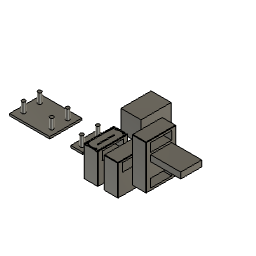
Scintillator Fittings (Autodesk Fusion 360 design; units mm, degrees)
Autodesk Fusion 360 part; units mm, degrees
note: some values were not read from the file. Set by a fixed rule: which sketch regions a step uses.
sketch "Sketch1" plane through (0, 0, 0) normal (0, 0, 1) x (1, 0, 0)
  line L0 (17.5, 37.5) -> (-17.5, 37.5)
  line L1 (-17.5, 37.5) -> (-17.5, -37.5)
  line L2 (-17.5, -37.5) -> (17.5, -37.5)
  line L3 (17.5, -37.5) -> (17.5, 37.5)
  line L4 (17.5, 37.5) -> (-17.5, -37.5) construction
  line L5 (-17.5, 37.5) -> (17.5, -37.5) construction
  dimension "d1" = 35
  dimension "d2" = 75
  constraint horizontal L0
  constraint perpendicular L0 L1
  constraint parallel L0 L2
  constraint parallel L1 L3
  constraint coincident L4 origin
  constraint coincident L5 origin
  measures "d1" distance of L1.end L2.end
  measures "d2" distance of L0.end L1.end
extrude "Extrude1" add sketch "Sketch1" along normal blind 5 makes body 1
sketch "Sketch2" plane through (0, 0, 5) normal (0, 0, 1) x (-1, 0, 0)
  line L0 (-17.5, 37.5) -> (-17.5, -37.5)
  line L1 (-17.5, -37.5) -> (17.5, -37.5)
  line L2 (17.5, -37.5) -> (17.5, 37.5)
  line L3 (17.5, 37.5) -> (-17.5, 37.5)
  line L4 (-17.5, -26.25) -> (17.5, -26.25)
  line L5 (17.5, -26.25) -> (17.5, 26.25)
  line L6 (17.5, 26.25) -> (-17.5, 26.25)
  line L7 (-17.5, 26.25) -> (-17.5, -26.25)
  line L8 (-17.5, -26.25) -> (17.5, 26.25) construction
  line L9 (17.5, -26.25) -> (-17.5, 26.25) construction
  dimension "d5" = 52.5
  constraint horizontal L4
  constraint perpendicular L4 L5
  constraint parallel L4 L6
  constraint parallel L5 L7
  constraint coincident L8 origin
  constraint coincident L9 origin
  measures "d5" distance of L4.end L5.end
extrude "Extrude2" add sketch "Sketch2" along normal blind 26 contours L0 L2 L3 L6 | L0 L1 L2 L4 bodies 1
sketch "Sketch3" plane through (0, -26.25, 0) normal (0, 1, 0) x (-1, 0, 0)
  line L0 (-17.5, 5) -> (17.5, 5)
  line L1 (17.5, 5) -> (17.5, 31)
  line L2 (17.5, 31) -> (-17.5, 31)
  line L3 (-17.5, 31) -> (-17.5, 5)
  line L4 (-17.5, 31) -> (17.5, 31)
  line L5 (17.5, 31) -> (17.5, 26)
  line L6 (17.5, 26) -> (-17.5, 26)
  line L7 (-17.5, 26) -> (-17.5, 31)
  dimension "d8" = 35
  dimension "d9" = 5
  constraint horizontal L4
  constraint vertical L5
  constraint horizontal L6
  constraint vertical L7
  constraint coincident L2.end L3.start
  measures "d8" distance of L2.end L1.end
  measures "d9" distance of L2.end L6.end
extrude "Extrude3" add sketch "Sketch3" along normal blind 52.5 contours L1 L2 L3 L4 L5 L6 L7 bodies 1
chamfer "Chamfer1" distance 1 angle 45 8 edges at (0, -37.5, 31) (17.5, 0, 31) (-17.5, 0, 31) (0, 37.5, 31) (17.5, 37.5, 15.5) (-17.5, 37.5, 15.5) (-17.5, -37.5, 15.5) (17.5, -37.5, 15.5) on bodies 1
sketch "Sketch4" plane through (0, 0, 31) normal (0, 0, 1) x (-1, 0, 0)
  line L0 (-16.5, 36.5) -> (-16.5, -36.5)
  line L1 (-16.5, -36.5) -> (16.5, -36.5)
  line L2 (16.5, -36.5) -> (16.5, 36.5)
  line L3 (16.5, 36.5) -> (-16.5, 36.5)
  line L4 (-16, 20) -> (-16, -20)
  line L5 (16, -20) -> (16, 20)
  line L6 (16, 20) -> (-16, -20) construction
  line L7 (-16, 20) -> (16, -20) construction
  circle A0 centre (0, -20) radius 16
  circle A1 centre (0, 20) radius 16
  dimension "d13" = 32
  dimension "d14" = 40
  dimension "d15" = 32
  dimension "d16" = 32
  constraint parallel L4 L5
  constraint coincident L6 origin
  constraint coincident L7 origin
  measures "d13" distance of L4.end L5.start
  measures "d14" distance of L4.start L4.end
  measures "d15" diameter of A0
  measures "d16" diameter of A1
extrude "Extrude4" cut sketch "Sketch4" against normal blind 2.5 contours L4 L5 A0 A1 | A1 | A0 bodies 1
sketch "Sketch5" plane through (0, 0, 28.5) normal (0, 0, 1) x (-1, 0, 0)
  arc A0 (16, 20) -> (-16, 20) centre (0, 20) ccw
  line L0 (-16, 20) -> (-16, -20)
  arc A1 (-16, -20) -> (16, -20) centre (0, -20) ccw
  line L1 (16, -20) -> (16, 20)
  circle A2 centre (0, -20) radius 1.25
  circle A3 centre (0, 20) radius 1.25
  line L2 (-1.25, -20) -> (-1.25, 20)
  line L3 (1.25, 20) -> (1.25, -20)
  line L4 (1.25, -20) -> (-1.25, 20) construction
  line L5 (-1.25, -20) -> (1.25, 20) construction
  dimension "d19" = 2.5
  dimension "d20" = 2.5
  dimension "d21" = 2.5
  dimension "d22" = 40
  constraint concentric A1 A2
  constraint concentric A0 A3
  constraint parallel L2 L3
  constraint coincident L4 origin
  constraint coincident L5 origin
  measures "d19" diameter of A2
  measures "d20" diameter of A3
  measures "d21" distance of L2.end L3.start
  measures "d22" distance of L2.start L2.end
extrude "Extrude5" cut sketch "Sketch5" against normal blind 2.5 contours A2 | A2 A3 L2 L3 | A3 bodies 1
sketch "Sketch6" plane through (0, 0, 31) normal (0, 0, 1) x (-1, 0, 0)
  line L0 (-16, -20) -> (-16, 20)
  arc A0 (16, 20) -> (-16, 20) centre (0, 20) ccw
  line L1 (16, 20) -> (16, -20)
  arc A1 (-16, -20) -> (16, -20) centre (0, -20) ccw
  line L2 (-16.5, 36.5) -> (-16.5, -36.5)
  line L3 (-16.5, -36.5) -> (16.5, -36.5)
  line L4 (16.5, -36.5) -> (16.5, 36.5)
  line L5 (16.5, 36.5) -> (-16.5, 36.5)
  line L6 (-15, -37.5) -> (15, -37.5)
  line L7 (15, -37.5) -> (15, 37.5)
  line L8 (15, 37.5) -> (-15, 37.5)
  line L9 (-15, 37.5) -> (-15, -37.5)
  line L10 (-15, -37.5) -> (15, 37.5) construction
  line L11 (15, -37.5) -> (-15, 37.5) construction
  line L12 (-10, 37.5) -> (10, 37.5)
  line L13 (10, 37.5) -> (10, -37.5)
  line L14 (10, -37.5) -> (-10, -37.5)
  line L15 (-10, -37.5) -> (-10, 37.5)
  line L16 (-10, 37.5) -> (10, -37.5) construction
  line L17 (10, 37.5) -> (-10, -37.5) construction
  dimension "d25" = 30
  dimension "d26" = 75
  dimension "d27" = 20
  dimension "d28" = 75
  constraint horizontal L6
  constraint perpendicular L6 L7
  constraint parallel L6 L8
  constraint parallel L7 L9
  constraint coincident L10 origin
  constraint coincident L11 origin
  constraint horizontal L12
  constraint perpendicular L12 L13
  constraint parallel L12 L14
  constraint parallel L13 L15
  constraint coincident L16 origin
  constraint coincident L17 origin
  measures "d25" distance of L7.end L8.end
  measures "d26" distance of L6.end L7.end
  measures "d27" distance of L13.end L14.end
  measures "d28" distance of L12.end L13.end
extrude "Extrude6" cut sketch "Sketch6" against normal blind 2.5 contours A1 L3 L9 L15 | A0 L5 L9 L15 | L3 L6 L9 L15 | L5 L8 L9 L15 | A1 L3 L7 L13 | A0 L5 L7 L13 | L3 L6 L7 L13 | L5 L7 L8 L13 bodies 1
chamfer "Chamfer2" distance 0.5 angle 45 8 edges at (-10, -34.495, 31) (10, -34.495, 31) (15, -31.0339, 31) (-15, -31.0339, 31) (-10, 34.495, 31) (-15, 31.0339, 31) (10, 34.495, 31) (15, 31.0339, 31) on bodies 1
sketch "Sketch7" plane through (0, 0, 0) normal (0, 0, 1) x (1, 0, 0)
  line L0 (32.5, 37.5) -> (67.5, 37.5)
  line L1 (67.5, 37.5) -> (67.5, -37.5)
  line L2 (67.5, -37.5) -> (32.5, -37.5)
  line L3 (32.5, -37.5) -> (32.5, 37.5)
  line L4 (32.5, 37.5) -> (67.5, -37.5) construction
  line L5 (67.5, 37.5) -> (32.5, -37.5) construction
  point P0 (50, 0)
  dimension "d32" = 35
  dimension "d33" = 75
  constraint horizontal L0
  constraint perpendicular L0 L1
  constraint parallel L0 L2
  constraint parallel L1 L3
  constraint coincident L4 P0
  constraint coincident L5 P0
  measures "d32" distance of L1.end L2.end
  measures "d33" distance of L0.end L1.end
extrude "Extrude7" add sketch "Sketch7" along normal blind 5 separate body makes body 2
sketch "Sketch8" plane through (0, 0, 5) normal (0, 0, 1) x (-1, 0, 0)
  line L0 (-32.5, 37.5) -> (-67.5, 37.5)
  line L1 (-67.5, 37.5) -> (-67.5, -37.5)
  line L2 (-67.5, -37.5) -> (-32.5, -37.5)
  line L3 (-32.5, -37.5) -> (-32.5, 37.5)
  line L4 (-67.5, -26.25) -> (-32.5, -26.25)
  line L5 (-32.5, -26.25) -> (-32.5, 26.25)
  line L6 (-32.5, 26.25) -> (-67.5, 26.25)
  line L7 (-67.5, 26.25) -> (-67.5, -26.25)
  line L8 (-67.5, -26.25) -> (-32.5, 26.25) construction
  line L9 (-32.5, -26.25) -> (-67.5, 26.25) construction
  point P0 (-50, 0)
  dimension "d36" = 52.5
  constraint horizontal L4
  constraint perpendicular L4 L5
  constraint parallel L4 L6
  constraint parallel L5 L7
  constraint coincident L8 P0
  constraint coincident L9 P0
  measures "d36" distance of L4.end L5.end
extrude "Extrude8" add sketch "Sketch8" along normal blind 26 contours L0 L1 L3 L6 | L1 L2 L3 L4 bodies 2
sketch "Sketch9" plane through (0, 26.25, 0) normal (0, -1, 0) x (1, 0, 0)
  line L0 (32.5, 5) -> (67.5, 5)
  line L1 (67.5, 5) -> (67.5, 31)
  line L2 (67.5, 31) -> (32.5, 31)
  line L3 (32.5, 31) -> (32.5, 5)
  line L4 (67.5, 31) -> (32.5, 31)
  line L5 (32.5, 31) -> (32.5, 26)
  line L6 (32.5, 26) -> (67.5, 26)
  line L7 (67.5, 26) -> (67.5, 31)
  dimension "d39" = 35
  dimension "d40" = 5
  constraint horizontal L4
  constraint vertical L5
  constraint horizontal L6
  constraint vertical L7
  constraint coincident L1.end L2.start
  measures "d39" distance of L1.end L2.end
  measures "d40" distance of L1.end L6.end
extrude "Extrude9" add sketch "Sketch9" along normal blind 52.5 contours L1 L2 L3 L4 L5 L6 L7 bodies 2
chamfer "Chamfer3" distance 1 angle 45 8 edges at (67.5, 0, 31) (67.5, -37.5, 15.5) (50, -37.5, 31) (50, 37.5, 31) (32.5, 0, 31) (67.5, 37.5, 15.5) (32.5, 37.5, 15.5) (32.5, -37.5, 15.5) on bodies 2
extrude "Extrude10" add 2 faces at (44.1667, 12.1667, 0) (-5.8333, 12.1667, 0) along direction (0, 0, -1) blind 45 on bodies 1 2 bodies 2 1
sketch "Sketch10" plane through (0, 0, -45) normal (0, 0, -1) x (1, 0, 0)
  line L0 (16.5, -37.5) -> (17.5, -36.5)
  line L1 (17.5, -36.5) -> (17.5, 36.5)
  line L2 (17.5, 36.5) -> (16.5, 37.5)
  line L3 (16.5, 37.5) -> (-16.5, 37.5)
  line L4 (-16.5, 37.5) -> (-17.5, 36.5)
  line L5 (-17.5, 36.5) -> (-17.5, -36.5)
  line L6 (-17.5, -36.5) -> (-16.5, -37.5)
  line L7 (-16.5, -37.5) -> (16.5, -37.5)
  circle A0 centre (0, 20) radius 5
  circle A1 centre (0, -20) radius 5
  dimension "d46" = 20
  dimension "d47" = 10
  dimension "d48" = 20
  dimension "d49" = 10
  dimension "d50" = 17.5
  dimension "d51" = 17.5
  measures "d46" distance of origin A0.centre
  measures "d47" diameter of A0
  measures "d48" distance of origin A1.centre
  measures "d49" diameter of A1
  measures "d50" distance of L1 A0.centre
  measures "d51" distance of L1 A1.centre
extrude "Extrude11" cut sketch "Sketch10" against normal blind 30 contours A0 | A1 bodies 1
sketch "Sketch11" plane through (0, 0, -45) normal (0, 0, -1) x (1, 0, 0)
  line L0 (32.5, -36.5) -> (33.5, -37.5)
  line L1 (33.5, -37.5) -> (66.5, -37.5)
  line L2 (66.5, -37.5) -> (67.5, -36.5)
  line L3 (67.5, -36.5) -> (67.5, 36.5)
  line L4 (67.5, 36.5) -> (66.5, 37.5)
  line L5 (66.5, 37.5) -> (33.5, 37.5)
  line L6 (33.5, 37.5) -> (32.5, 36.5)
  line L7 (32.5, 36.5) -> (32.5, -36.5)
  circle A0 centre (50, 20) radius 5
  circle A1 centre (50, -20) radius 5
  dimension "d54" = 10
  dimension "d55" = 10
  measures "d54" diameter of A0
  measures "d55" diameter of A1
extrude "Extrude12" cut sketch "Sketch11" against normal blind 30 contours A0 | A1 bodies 2
sketch "Sketch12" plane through (0, 0, 0) normal (0, 0, 1) x (1, 0, 0)
  line L0 (-25, 32.5) -> (-55, 32.5)
  line L1 (-55, 32.5) -> (-55, -32.5)
  line L2 (-55, -32.5) -> (-25, -32.5)
  line L3 (-25, -32.5) -> (-25, 32.5)
  line L4 (-25, 32.5) -> (-55, -32.5) construction
  line L5 (-55, 32.5) -> (-25, -32.5) construction
  point P0 (-40, 0)
  dimension "d58" = 30
  dimension "d59" = 65
  constraint horizontal L0
  constraint perpendicular L0 L1
  constraint parallel L0 L2
  constraint parallel L1 L3
  constraint coincident L4 P0
  constraint coincident L5 P0
  measures "d58" distance of L1.end L2.end
  measures "d59" distance of L0.end L1.end
extrude "Extrude13" add sketch "Sketch12" along normal blind 5 separate body makes body 3
sketch "Sketch13" plane through (0, 0, 5) normal (0, 0, 1) x (-1, 0, 0)
  line L0 (25, 32.5) -> (25, -32.5)
  line L1 (25, -32.5) -> (55, -32.5)
  line L2 (55, -32.5) -> (55, 32.5)
  line L3 (55, 32.5) -> (25, 32.5)
  line L4 (40, 0) -> (40, -20)
  circle A0 centre (40, -20) radius 4.5
  line L5 (40, 0) -> (40, 20)
  circle A1 centre (40, 20) radius 4.5
  dimension "d62" = 20
  dimension "d63" = 9
  dimension "d64" = 20
  dimension "d65" = 9
  constraint vertical L4
  constraint coincident L4.end A0.centre
  constraint parallel L4 L5
  constraint coincident L5.end A1.centre
  measures "d62" distance of L4.start L4.end
  measures "d63" diameter of A0
  measures "d64" distance of L4.start L5.end
  measures "d65" diameter of A1
extrude "Extrude14" add sketch "Sketch13" along normal blind 25 contours A0 | A1 bodies 3
sketch "Sketch14" plane through (0, 0, 0) normal (0, 0, 1) x (1, 0, 0)
  line L0 (137.5, 37.5) -> (102.5, 37.5)
  line L1 (102.5, 37.5) -> (102.5, -37.5)
  line L2 (102.5, -37.5) -> (137.5, -37.5)
  line L3 (137.5, -37.5) -> (137.5, 37.5)
  line L4 (137.5, 37.5) -> (102.5, -37.5) construction
  line L5 (102.5, 37.5) -> (137.5, -37.5) construction
  point P0 (120, 0)
  dimension "d68" = 35
  dimension "d69" = 75
  constraint horizontal L0
  constraint perpendicular L0 L1
  constraint parallel L0 L2
  constraint parallel L1 L3
  constraint coincident L4 P0
  constraint coincident L5 P0
  measures "d68" distance of L1.end L2.end
  measures "d69" distance of L0.end L1.end
extrude "Extrude15" add sketch "Sketch14" along normal blind 110 separate body makes body 4
sketch "Sketch15" plane through (102.5, 0, 0) normal (-1, 0, 0) x (0, -1, 0)
  line L0 (-37.5, 0) -> (37.5, 0)
  line L1 (37.5, 0) -> (37.5, 110)
  line L2 (37.5, 110) -> (-37.5, 110)
  line L3 (-37.5, 110) -> (-37.5, 0)
  line L4 (-37.5, 110) -> (0, 110)
  line L5 (0, 110) -> (0, 93.5)
  line L6 (26.25, 104) -> (-26.25, 104)
  line L7 (-26.25, 104) -> (-26.25, 83)
  line L8 (-26.25, 83) -> (26.25, 83)
  line L9 (26.25, 83) -> (26.25, 104)
  line L10 (26.25, 104) -> (-26.25, 83) construction
  line L11 (-26.25, 104) -> (26.25, 83) construction
  line L12 (-37.5, 0) -> (0, 0)
  line L13 (0, 0) -> (0, 16.5)
  line L14 (26.25, 27) -> (-26.25, 27)
  line L15 (-26.25, 27) -> (-26.25, 6)
  line L16 (-26.25, 6) -> (26.25, 6)
  line L17 (26.25, 6) -> (26.25, 27)
  line L18 (26.25, 27) -> (-26.25, 6) construction
  line L19 (-26.25, 27) -> (26.25, 6) construction
  point P0 (0, 93.5)
  point P1 (0, 16.5)
  dimension "d72" = 37.5
  dimension "d74" = 16.5
  dimension "d75" = 52.5
  dimension "d76" = 21
  dimension "d77" = 37.5
  dimension "d78" = 16.5
  dimension "d79" = 52.5
  dimension "d80" = 21
  constraint coincident L2.end L3.start
  constraint perpendicular L3 L4
  constraint perpendicular L4 L5
  constraint horizontal L6
  constraint perpendicular L6 L7
  constraint parallel L6 L8
  constraint parallel L7 L9
  constraint coincident L10 P0
  constraint coincident L11 P0
  constraint coincident P0 L5.end
  constraint coincident L0.start L3.end
  constraint perpendicular L3 L12
  constraint perpendicular L12 L13
  constraint horizontal L14
  constraint perpendicular L14 L15
  constraint parallel L14 L16
  constraint parallel L15 L17
  constraint coincident L18 P1
  constraint coincident L19 P1
  constraint coincident P1 L13.end
  measures "d72" distance of L2.end L4.end
  measures "d74" distance of L4.end P0
  measures "d75" distance of L7.end L8.end
  measures "d76" distance of L6.end L7.end
  measures "d77" distance of L0.start L12.end
  measures "d78" distance of L12.end P1
  measures "d79" distance of L15.end L16.end
  measures "d80" distance of L14.end L15.end
extrude "Extrude16" cut sketch "Sketch15" against normal blind 35 contours L6 L7 L8 L9 | L14 L15 L16 L17 bodies 4
chamfer "Chamfer4" distance 1 angle 45 12 edges at (102.5, -37.5, 55) (102.5, 0, 110) (102.5, 37.5, 55) (120, 37.5, 110) (137.5, 0, 110) (120, -37.5, 110) (102.5, 0, 0) (120, 37.5, 0) (137.5, 37.5, 55) (137.5, 0, 0) (137.5, -37.5, 55) (120, -37.5, 0) on bodies 4
sketch "Sketch16" plane through (137.5, 0, 0) normal (1, 0, 0) x (0, 1, 0)
  line L0 (-26.25, 104) -> (26.25, 104)
  line L1 (26.25, 104) -> (26.25, 83)
  line L2 (26.25, 83) -> (-26.25, 83)
  line L3 (-26.25, 83) -> (-26.25, 104)
  line L4 (-26.25, 27) -> (26.25, 27)
  line L5 (26.25, 27) -> (26.25, 6)
  line L6 (26.25, 6) -> (-26.25, 6)
  line L7 (-26.25, 6) -> (-26.25, 27)
  line L8 (-36.5, 1) -> (36.5, 1)
  line L9 (36.5, 1) -> (36.5, 109)
  line L10 (36.5, 109) -> (-36.5, 109)
  line L11 (-36.5, 109) -> (-36.5, 1)
  line L12 (-26.25, 78) -> (26.25, 78)
  line L13 (26.25, 78) -> (26.25, 63)
  line L14 (26.25, 63) -> (-26.25, 63)
  line L15 (-26.25, 63) -> (-26.25, 78)
  dimension "d84" = 5
  dimension "d85" = 52.5
  dimension "d86" = 15
  constraint horizontal L12
  constraint vertical L13
  constraint horizontal L14
  constraint vertical L15
  measures "d84" distance of L2.end L12.start
  measures "d85" distance of L12.start L12.end
  measures "d86" distance of L12.start L14.end
extrude "Extrude17" add sketch "Sketch16" along normal blind 75 contours L12 L13 L14 L15 bodies 4
sketch "Sketch17" plane through (0, 0, 0) normal (0, 0, 1) x (1, 0, 0)
  line L0 (-200, 40) -> (-100, 40)
  line L1 (-100, 40) -> (-100, -40)
  line L2 (-100, -40) -> (-200, -40)
  line L3 (-200, -40) -> (-200, 40)
  line L4 (-200, 40) -> (-100, -40) construction
  line L5 (-100, 40) -> (-200, -40) construction
  point P0 (-150, 0)
  dimension "d89" = 100
  dimension "d90" = 80
  constraint horizontal L0
  constraint perpendicular L0 L1
  constraint parallel L0 L2
  constraint parallel L1 L3
  constraint coincident L4 P0
  constraint coincident L5 P0
  measures "d89" distance of L1.end L2.end
  measures "d90" distance of L0.end L1.end
extrude "Extrude18" add sketch "Sketch17" along normal blind 5 separate body makes body 5
sketch "Sketch18" plane through (0, 0, 5) normal (0, 0, 1) x (-1, 0, 0)
  line L0 (200, 40) -> (100, 40)
  line L1 (100, 40) -> (100, -40)
  line L2 (100, -40) -> (200, -40)
  line L3 (200, -40) -> (200, 40)
  line L4 (100, 0) -> (115, 0)
  line L5 (115, 0) -> (115, -20)
  line L6 (115, -20) -> (100, -20)
  line L7 (100, -20) -> (100, 0)
  circle A0 centre (115, -20) radius 4.5
  line L8 (100, 0) -> (115, 0)
  line L9 (115, 0) -> (115, 20)
  line L10 (115, 20) -> (100, 20)
  line L11 (100, 20) -> (100, 0)
  circle A1 centre (115, 20) radius 4.5
  dimension "d93" = 15
  dimension "d94" = 20
  dimension "d95" = 9
  dimension "d96" = 20
  dimension "d97" = 9
  constraint horizontal L4
  constraint vertical L5
  constraint horizontal L6
  constraint vertical L7
  constraint midpoint L1 L4.start
  constraint coincident L5.end L6.start
  constraint horizontal L8
  constraint vertical L9
  constraint horizontal L10
  constraint vertical L11
  constraint coincident L9.end L10.start
  measures "d93" distance of L4.start L4.end
  measures "d94" distance of L4.start L6.end
  measures "d95" diameter of A0
  measures "d96" distance of L4.start L10.end
  measures "d97" diameter of A1
extrude "Extrude19" add sketch "Sketch18" along normal blind 25 contours L9 L10 A1 | L9 L10 A1 | L5 L6 A0 | L5 L6 A0 bodies 5
sketch "Sketch19" plane through (0, 0, 5) normal (0, 0, 1) x (-1, 0, 0)
  circle A0 centre (115, 20) radius 4.5
  circle A1 centre (115, -20) radius 4.5
  line L0 (200, 40) -> (100, 40)
  line L1 (100, 40) -> (100, -40)
  line L2 (100, -40) -> (200, -40)
  line L3 (200, -40) -> (200, 40)
  line L4 (200, 0) -> (185, 0)
  line L5 (185, 0) -> (185, 20)
  line L6 (185, 20) -> (200, 20)
  line L7 (200, 20) -> (200, 0)
  line L8 (200, 0) -> (185, 0)
  line L9 (185, 0) -> (185, -20)
  line L10 (185, -20) -> (200, -20)
  line L11 (200, -20) -> (200, 0)
  circle A2 centre (185, -20) radius 4.5
  circle A3 centre (185, 20) radius 4.5
  dimension "d100" = 15
  dimension "d101" = 20
  dimension "d102" = 20
  dimension "d103" = 9
  dimension "d104" = 9
  constraint horizontal L4
  constraint vertical L5
  constraint horizontal L6
  constraint vertical L7
  constraint midpoint L3 L4.start
  constraint horizontal L8
  constraint vertical L9
  constraint horizontal L10
  constraint vertical L11
  constraint coincident L9.end L10.start
  constraint coincident L5.end L6.start
  measures "d100" distance of L4.start L4.end
  measures "d101" distance of L4.start L6.end
  measures "d102" distance of L4.start L10.end
  measures "d103" diameter of A2
  measures "d104" diameter of A3
extrude "Extrude20" add sketch "Sketch19" along normal blind 25 contours L5 L6 A3 | L5 L6 A3 | L9 L10 A2 | L9 L10 A2 bodies 5
sketch "Sketch20" plane through (0, 0, 0) normal (0, 0, 1) x (1, 0, 0)
  line L0 (25, 62.5) -> (-25, 62.5)
  line L1 (-25, 62.5) -> (-25, 137.5)
  line L2 (-25, 137.5) -> (25, 137.5)
  line L3 (25, 137.5) -> (25, 62.5)
  line L4 (25, 62.5) -> (-25, 137.5) construction
  line L5 (-25, 62.5) -> (25, 137.5) construction
  point P0 (0, 100)
  dimension "d107" = 50
  dimension "d108" = 75
  constraint horizontal L0
  constraint perpendicular L0 L1
  constraint parallel L0 L2
  constraint parallel L1 L3
  constraint coincident L4 P0
  constraint coincident L5 P0
  measures "d107" distance of L1.end L2.end
  measures "d108" distance of L0.end L1.end
extrude "Extrude21" add sketch "Sketch20" along normal blind 52.5 separate body makes body 6
sketch "Sketch21" plane through (0, 0, 0) normal (0, 0, -1) x (1, 0, 0)
  line L0 (-25, -137.5) -> (25, -137.5)
  line L1 (25, -137.5) -> (25, -62.5)
  line L2 (25, -62.5) -> (-25, -62.5)
  line L3 (-25, -62.5) -> (-25, -137.5)
  line L4 (0, -100) -> (0, -80)
  line L5 (0, -100) -> (0, -120)
  circle A0 centre (0, -80) radius 5
  circle A1 centre (0, -120) radius 5
  dimension "d111" = 20
  dimension "d112" = 20
  dimension "d113" = 10
  dimension "d114" = 10
  constraint vertical L4
  constraint parallel L4 L5
  constraint coincident L4.end A0.centre
  constraint coincident L5.end A1.centre
  measures "d111" distance of L4.start L4.end
  measures "d112" distance of L4.start L5.end
  measures "d113" diameter of A0
  measures "d114" diameter of A1
extrude "Extrude22" cut sketch "Sketch21" against normal blind 30 contours A0 | A1 bodies 6
